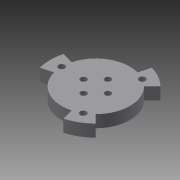
# Autodesk Inventor part: Hub_Adapter_Acryllic
Saved by Autodesk Inventor 2015 SP1 (Build 190203100, 203)
## iProperties
Created: 2016-04-07
Part Number: Hub_Adapter_Acryllic
Material: Generic
Document SubType Name: Modeling
Designer: Ethan
Density: 1 g/cm^3
Appearance: Default
Author: Ethan
Autodesk Inventor part; units mm, degrees
ref_plane "YZ Plane" through (0, 0, 0) normal (1, 0, 0) x (0, 1, 0)
ref_plane "XZ Plane" through (0, 0, 0) normal (0, 1, 0) x (-1, 0, 0)
ref_plane "XY Plane" through (0, 0, 0) normal (0, 0, 1) x (1, 0, 0)
sketch "Sketch1" plane through (0, 0, 0) normal (0, 1, 0) x (-1, 0, 0)
  line L0 (17.1742, 4.6018) -> (23.0011, 6.1631)
  line L1 (17.1742, -4.6018) -> (23.0011, -6.1631)
  circle A0 centre (17.78, 0) radius 1.651
  line L2 (-12.5724, 12.5724) -> (-16.838, 16.838)
  line L3 (-4.6018, 17.1742) -> (-6.1631, 23.0011)
  circle A1 centre (-8.89, 15.3979) radius 1.651
  line L4 (-4.6018, -17.1742) -> (-6.1631, -23.0011)
  line L5 (-12.5724, -12.5724) -> (-16.838, -16.838)
  circle A2 centre (-8.89, -15.3979) radius 1.651
  arc A3 (-6.1631, 23.0011) -> (-16.838, 16.838) centre (0, 0) ccw
  arc A4 (-16.838, -16.838) -> (-6.1631, -23.0011) centre (0, 0) ccw
  arc A5 (23.0011, -6.1631) -> (23.0011, 6.1631) centre (0, 0) ccw
  arc A6 (-12.5724, 12.5724) -> (-12.5724, -12.5724) centre (0, 0) ccw
  arc A7 (-4.6018, -17.1742) -> (17.1742, -4.6018) centre (0, 0) ccw
  arc A8 (17.1742, 4.6018) -> (-4.6018, 17.1742) centre (0, 0) ccw
  circle A9 centre (6.35, 0) radius 1.5875
  circle A10 centre (0, 6.35) radius 1.5875
  circle A11 centre (-6.35, 0) radius 1.5875
  circle A12 centre (0, -6.35) radius 1.5875
  dimension "d3" = 3.302
  dimension "d9" = 3.175
  dimension "d12" = 360
  dimension "d15" = 6.35
  constraints: 13 centre point, 13 point on circle, 12 end point, 2 coincident, 34 other
  measures "d3" diameter of A0
  measures "d9" diameter of A9
  measures "d15" distance of A11.centre point (0, 0)
extrude "Extrusion1" add sketch "Sketch1" along normal blind 6.35
body "Solid1"
